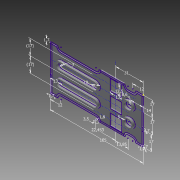
# Autodesk Inventor part: Top_V4
Saved by Autodesk Inventor 2016 (Build 200138000, 138)
## iProperties
Created: 2015-06-18
Part Number: Top_V4
Material: Generic
Document SubType Name: Modeling
Designer: Openlab
Density: 1 g/cm^3
Appearance: Default
Author: Openlab
Autodesk Inventor part; units mm, degrees
ref_plane "YZ Plane" through (0, 0, 0) normal (1, 0, 0) x (0, 1, 0)
ref_plane "XZ Plane" through (0, 0, 0) normal (0, 1, 0) x (-1, 0, 0)
ref_plane "XY Plane" through (0, 0, 0) normal (0, 0, 1) x (1, 0, 0)
sketch "Sketch1" plane through (0, 0, 0) normal (0, 1, 0) x (-1, 0, 0)
  line L0 (37.5, -2.25) -> (24.5, -2.25)
  line L1 (24.5, -2.25) -> (24.5, -14.75)
  line L2 (24.5, -14.75) -> (37.5, -14.75)
  line L3 (37.5, -14.75) -> (37.5, -2.25)
  line L4 (56.9183, -8.5) -> (8.3915, -8.5) construction
  line L5 (0, -17) -> (105, -17) construction
  line L6 (0, 0) -> (0, -51)
  line L7 (0, -34) -> (105, -34) construction
  line L8 (105, -51) -> (105, 0)
  line L9 (31, 19) -> (31, -51) construction
  line L10 (56.8064, -25.5) -> (17, -25.5) construction
  line L11 (24.5, -19.25) -> (24.5, -31.75)
  line L12 (37.5, -19.25) -> (24.5, -19.25)
  line L13 (37.5, -31.75) -> (37.5, -19.25)
  line L14 (24.5, -31.75) -> (37.5, -31.75)
  line L15 (24.5, -36.25) -> (24.5, -48.75)
  line L16 (37.5, -36.25) -> (24.5, -36.25)
  line L17 (37.5, -48.75) -> (37.5, -36.25)
  line L18 (24.5, -48.75) -> (37.5, -48.75)
  line L19 (56.3008, -42.5) -> (16.5498, -42.5) construction
  arc A0 (53.453, -12) -> (53.453, -22) centre (53.453, -17) ccw
  arc A1 (92, -22) -> (92, -12) centre (92, -17) ccw
  arc A2 (53.453, -29) -> (53.453, -39) centre (53.453, -34) ccw
  arc A3 (92, -39) -> (92, -29) centre (92, -34) ccw
  line L20 (53.453, -12) -> (92, -12)
  line L21 (53.453, -22) -> (92, -22)
  line L22 (53.453, -29) -> (92, -29)
  line L23 (53.453, -39) -> (92, -39)
  arc A4 (15.9, -39) -> (15.9, -29) centre (15.9, -34) ccw
  line L24 (103.3, -49.3) -> (103.3, -1.7)
  line L25 (1.7, -1.7) -> (1.7, -49.3)
  arc A5 (14, -29) -> (14, -39) centre (14, -34) ccw
  arc A6 (14, -12) -> (14, -22) centre (14, -17) ccw
  line L26 (15.9, -39) -> (14, -39)
  line L27 (14, -29) -> (15.9, -29)
  line L28 (14, -22) -> (15.9, -22)
  line L29 (15.9, -12) -> (14, -12)
  arc A7 (15.9, -22) -> (15.9, -12) centre (15.9, -17) ccw
  arc A8 (96.5, -51) -> (93, -47.5) centre (93, -51) ccw
  arc A9 (53.453, -47.5) -> (49.953, -51) centre (53.453, -51) ccw
  arc A10 (98.02, -49.3) -> (93, -45.7) centre (93, -51) ccw
  line L30 (93, -45.7) -> (53.453, -45.7)
  line L31 (96.5, -51) -> (105, -51)
  line L32 (93, -47.5) -> (53.453, -47.5)
  line L33 (105, -49.3) -> (98.02, -49.3)
  arc A11 (53.453, -45.7) -> (48.433, -49.3) centre (53.453, -51) ccw
  arc A12 (48.433, -1.7) -> (53.453, -5.3) centre (53.453, 0) ccw
  arc A13 (49.953, 0) -> (53.453, -3.5) centre (53.453, 0) ccw
  line L34 (93, -3.5) -> (53.453, -3.5)
  line L35 (93, -5.3) -> (53.453, -5.3)
  line L36 (98.02, -1.7) -> (105, -1.7)
  line L37 (105, 0) -> (96.5, 0)
  arc A14 (93, -3.5) -> (96.5, 0) centre (93, 0) ccw
  arc A15 (93, -5.3) -> (98.02, -1.7) centre (93, 0) ccw
  arc A16 (20.65, -51) -> (17.15, -47.5) centre (17.15, -51) ccw
  arc A17 (12, -47.5) -> (8.5, -51) centre (12, -51) ccw
  line L38 (17.15, -45.7) -> (12, -45.7)
  line L39 (17.15, -47.5) -> (12, -47.5)
  arc A18 (12, -45.7) -> (6.98, -49.3) centre (12, -51) ccw
  arc A19 (22.17, -49.3) -> (17.15, -45.7) centre (17.15, -51) ccw
  line L40 (48.433, -49.3) -> (22.17, -49.3)
  line L41 (6.98, -49.3) -> (0, -49.3)
  line L42 (0, -51) -> (8.5, -51)
  line L43 (20.65, -51) -> (49.953, -51)
  line L44 (17.15, -5.3) -> (12, -5.3)
  line L45 (17.15, -3.5) -> (12, -3.5)
  arc A20 (8.5, 0) -> (12, -3.5) centre (12, 0) ccw
  arc A21 (17.15, -3.5) -> (20.65, 0) centre (17.15, 0) ccw
  arc A22 (6.98, -1.7) -> (12, -5.3) centre (12, 0) ccw
  arc A23 (17.15, -5.3) -> (22.17, -1.7) centre (17.15, 0) ccw
  line L46 (49.953, 0) -> (20.65, 0)
  line L47 (8.5, 0) -> (0, 0)
  line L48 (0, -1.7) -> (6.98, -1.7)
  line L49 (22.17, -1.7) -> (48.433, -1.7)
  line L50 (48.433, -49.3) -> (48.433, -51)
  line L51 (22.17, -49.3) -> (22.17, -51)
  line L52 (48.433, -1.7) -> (48.433, 0)
  line L53 (22.17, -1.7) -> (22.17, 0)
  line L54 (103.3, -35.85) -> (105, -35.85)
  line L55 (105, -32.15) -> (103.3, -32.15)
  line L56 (1.7, -32.15) -> (0, -32.15)
  line L57 (0, -35.85) -> (1.7, -35.85)
  arc A24 (92, -20.5) -> (92, -13.5) centre (92, -17) ccw
  arc A25 (53.453, -13.5) -> (53.453, -20.5) centre (53.453, -17) ccw
  arc A26 (92, -37.5) -> (92, -30.5) centre (92, -34) ccw
  arc A27 (53.453, -30.5) -> (53.453, -37.5) centre (53.453, -34) ccw
  arc A28 (15.9, -20.5) -> (15.9, -13.5) centre (15.9, -17) ccw
  arc A29 (14, -13.5) -> (14, -20.5) centre (14, -17) ccw
  arc A30 (15.9, -37.5) -> (15.9, -30.5) centre (15.9, -34) ccw
  arc A31 (14, -30.5) -> (14, -37.5) centre (14, -34) ccw
  line L58 (92, -13.5) -> (53.453, -13.5)
  line L59 (92, -20.5) -> (53.453, -20.5)
  line L60 (92, -30.5) -> (53.453, -30.5)
  line L61 (92, -37.5) -> (53.453, -37.5)
  line L62 (15.9, -30.5) -> (14, -30.5)
  line L63 (15.9, -37.5) -> (14, -37.5)
  line L64 (15.9, -20.5) -> (14, -20.5)
  line L65 (15.9, -13.5) -> (14, -13.5)
  point P0 (31, -42.5)
  point P1 (31, -25.5)
  point P2 (31, -8.5)
  dimension "d0" = 13
  dimension "d1" = 12.5
  dimension "d12" = 17
  dimension "d18" = 105
  dimension "d20" = 17
  dimension "d22" = 17
  dimension "d32" = 10
  dimension "d33" = 1.7
  dimension "d34" = 1.7
  dimension "d38" = 5
  dimension "d43" = 1.7
  dimension "d44" = 1.7
  dimension "d45" = 17
  dimension "d50" = 17
  dimension "d51" = 12
  dimension "d52" = 13
  dimension "d56" = 12
  dimension "d67" = 3.5
  dimension "d68" = 1.8
  dimension "d72" = 14
  dimension "d73" = 22.453
  dimension "d74" = 13.85
  dimension "d75" = 31
  dimension "d76" = 8.6
  dimension "d77" = 3.7
  dimension "d78" = 7
  constraints: 132 end point, 64 point on circle, 52 point on line, 32 centre point, 29 tangent, 27 equal radius, 20 perpendicular, 17 coincident, 15 collinear, 15 parallel, 12 horizontal, 9 vertical alignment, 7 horizontal alignment, 1 vertical, 9 other
  measures "d0" distance of L2.end L1.end
  measures "d1" distance of L0.end L1.end
  measures "d12" distance between parallel lines of L10 L4
  measures "d18" distance between parallel lines of L6 L8
  measures "d20" distance between parallel lines of L19 L10
  measures "d22" distance between parallel lines of L5 L7
  measures "d32" diameter of A0
  measures "d33" distance between parallel lines of L6 L25
  measures "d34" distance between parallel lines of L8 L24
  measures "d38" radius of A4
  measures "d43" distance between parallel lines of L37 L36
  measures "d44" distance between parallel lines of L41 L42
  measures "d45" distance between parallel lines of L7 L42
  measures "d50" distance between parallel lines of L47 L5
  measures "d51" distance from line of A8.centre L8
  measures "d52" distance from line of L8 A3.centre
  measures "d56" distance from line of L6 A22.centre
  measures "d67" radius of A9
  measures "d68" radial gap between concentric circles of A9 A11
  measures "d72" distance of L5.start A6.centre
  measures "d73" distance from line of A9.centre L9
  measures "d74" distance from line of A16.centre L9
  measures "d75" distance between parallel lines of L6 L9
  measures "d76" distance from line of L1 A7.centre
  measures "d77" distance between parallel lines of L57 L56
  measures "d78" diameter of A24
extrude "Extrusion1" add sketch "Sketch1" along normal blind 1.5 contours L56 L25 L57 L6 | L48 A22 L44 A23 L49 A12 L35 A15 L36 L24 L33 A10 L30 A11 L40 A19 L38 A18 L41 L25 | L46 L52 L49 L53 | L40 L50 L43 L51 | L55 L8 L54 L24 | L20 A1 L21 A0 | L22 A3 L23 A2 | L26 A5 L27 A4 | L29 A7 L28 A6
chamfer "Chamfer1" distance 0.5 angle 45 32 edges at (-31, 0, -36.25) (-37.5, 0, -42.5) (-24.5, 0, -42.5) (-31, 0, -48.75) (-31, 0, -31.75) (-37.5, 0, -25.5) (-31, 0, -19.25) (-24.5, 0, -25.5) (-31, 0, -14.75) (-37.5, 0, -8.5) (-31, 0, -2.25) (-24.5, 0, -8.5) (-73.2265, 1.5, -45.7) (-96.0887, 1.5, -46.693) (-50.3643, 1.5, -46.693) (-100.66, 1.5, -49.3) (-103.3, 1.5, -42.575) (-103.3, 1.5, -16.925) (-100.66, 1.5, -1.7) (-96.0887, 1.5, -4.307) (-73.2265, 1.5, -5.3) (-50.3643, 1.5, -4.307) (-20.2387, 1.5, -4.307) (-14.575, 1.5, -5.3) (-8.9113, 1.5, -4.307) (-20.2387, 1.5, -46.693) (-14.575, 1.5, -45.7) (-8.9113, 1.5, -46.693) (-4.34, 1.5, -49.3) (-1.7, 1.5, -42.575) (-1.7, 1.5, -16.925) (-4.34, 1.5, -1.7)
extrude "Extrusion3" add sketch "Sketch1" against normal blind 2.75 contours L20 A1 L21 A0 | L22 A3 L23 A2 | L26 A5 L27 A4 | L29 A7 L28 A6
body "Solid1"
